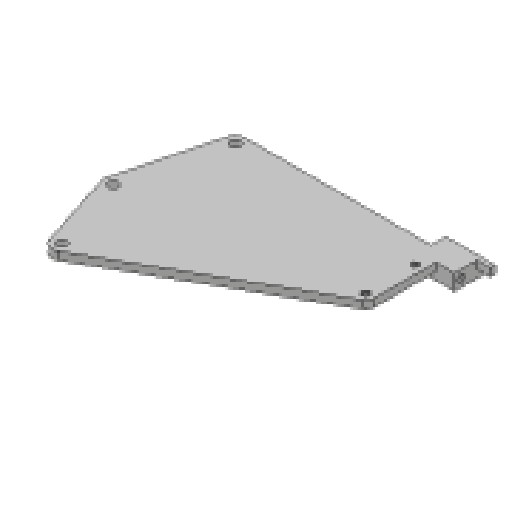
# Autodesk Inventor part: intakeSlidesWheelHolder
Saved by Autodesk Inventor 2023 (Build 270158000, 158)
## iProperties
Created: 2022-11-03
Part Number: intakeSlidesWheelHolder
Material: Generic
Document SubType Name: Modeling
Designer: deli
Density: 1 g/cm^3
Appearance: Default
Author: deli
Autodesk Inventor part; units mm, degrees
ref_plane "YZ Plane" through (0, 0, 0) normal (1, 0, 0) x (0, 1, 0)
ref_plane "XZ Plane" through (0, 0, 0) normal (0, 1, 0) x (-1, 0, 0)
ref_plane "XY Plane" through (0, 0, 0) normal (0, 0, 1) x (1, 0, 0)
sketch "Sketch1" plane through (0, 0, 0) normal (0, 1, 0) x (-1, 0, 0)
  circle A0 centre (23.0548, 41.1652) radius 1.5
  circle A1 centre (23.0548, 21.1652) radius 1.5
  arc A2 (26.5548, 41.1652) -> (19.5548, 41.1652) centre (23.0548, 41.1652) ccw
  line L0 (26.5548, 41.1652) -> (26.5548, 11.1652)
  line L1 (101.8798, 11.1652) -> (12.0548, 11.1652)
  line L2 (19.5548, 16.1652) -> (19.5548, 41.1652)
  line L3 (12.0548, 11.1652) -> (12.0548, 16.1652)
  line L4 (12.0548, 16.1652) -> (19.5548, 16.1652)
  circle A3 centre (112.0548, 54.1652) radius 2
  circle A4 centre (112.0548, 54.1652) radius 25 construction
  circle A5 centre (101.8798, 15.1652) radius 2
  circle A6 centre (101.8798, 85.1652) radius 2
  arc A7 (101.8798, 11.1652) -> (105.7503, 14.1554) centre (101.8798, 15.1652) ccw
  arc A8 (115.9253, 53.1554) -> (115.8554, 55.4126) centre (112.0548, 54.1652) ccw
  arc A9 (105.6804, 86.4126) -> (99.9109, 88.6471) centre (101.8798, 85.1652) ccw
  line L5 (105.7503, 14.1554) -> (115.9253, 53.1554)
  line L6 (115.8554, 55.4126) -> (105.6804, 86.4126)
  line L7 (21.332, 44.2118) -> (99.9109, 88.6471)
  line L8 (12.0548, 11.1652) -> (26.5548, 11.1652)
  line L9 (26.5548, 11.1652) -> (26.5548, 5.1652)
  line L10 (26.5548, 5.1652) -> (11.2902, 5.1652)
  line L11 (12.0548, 7.1652) -> (12.0548, 11.1652)
  line L12 (11.2902, 5.1652) -> (6.7902, 5.1652)
  line L13 (6.7902, 5.1652) -> (6.7902, 7.1652)
  line L14 (6.7902, 7.1652) -> (12.0548, 7.1652)
  point P0 (0, 0)
  dimension "d0" = 3
  dimension "d1" = 2
  dimension "d2" = 20
  dimension "d3" = 10
  dimension "d20" = 11
  dimension "d28" = 4
  dimension "d29" = 85.5
  dimension "d30" = 3.5
  dimension "d32" = 5
  dimension "d33" = 50
  dimension "d34" = 4
  dimension "d35" = 75.325
  dimension "d36" = 75.325
  dimension "d39" = 8
  dimension "d40" = 39
  dimension "d42" = 31
  dimension "d43" = 11
  dimension "d58" = 2
  dimension "d59" = 4.5
  constraints: 30 end point, 10 centre point, 9 point on circle, 9 tangent, 5 coincident, 4 equal radius, 4 horizontal, 4 perpendicular, 3 parallel, 2 collinear, 2 point on line, 1 vertical
  measures "d0" diameter of A0
  measures "d1" radial gap between concentric circles of A2 A0
  measures "d2" distance of A0.centre A1.centre
  measures "d3" distance from line of L1 A1.centre
  measures "d20" distance from line of A1.centre L3
  measures "d28" diameter of A3
  measures "d29" distance from line of L0 A3.centre
  measures "d30" distance from line of A1.centre L0
  measures "d32" distance of L1.end L3.end
  measures "d33" diameter of A4
  measures "d34" diameter of A5
  measures "d35" distance from line of L0 A5.centre
  measures "d36" distance from line of A6.centre L0
  measures "d39" diameter of A7
  measures "d40" vertical distance of A3.centre A5.centre
  measures "d42" vertical distance of A6.centre A3.centre
  measures "d43" distance between parallel lines of L4 L10
  measures "d58" distance of L12.end L13.end
  measures "d59" distance of L10.end L12.end
extrude "Extrusion1" add sketch "Sketch1" along normal blind 3.175
sketch "Sketch2" plane through (0, 3.175, 0) normal (0, 1, 0) x (1, 0, 0)
  line L0 (-19.5548, -16.1652) -> (-12.0548, -16.1652) projected
  line L1 (-6.7902, -5.1652) -> (-26.5548, -5.1652) projected
  line L2 (-12.0548, -16.1652) -> (-26.5548, -16.1652)
  line L3 (-26.5548, -16.1652) -> (-26.5548, -5.1652)
  line L4 (-26.5548, -5.1652) -> (-12.0548, -5.1652)
  line L5 (-12.0548, -5.1652) -> (-12.0548, -16.1652)
  point P0 (0, 0)
  point P1 (-12.0548, -1.1652)
  point P2 (-12.0548, -1.1652)
  constraints: 8 end point, 2 parallel, 1 horizontal, 1 perpendicular, 1 other
extrude "Extrusion2" add sketch "Sketch2" against normal blind 6.35
thread "Thread1" size "M3x0.5" class "6H" standard "ANSI Metric M Profile" full length
thread "Thread3" size "M3x0.5" class "6H" standard "ANSI Metric M Profile" full length
sketch "Sketch5" plane through (-12.0548, 3.175, 16.1652) normal (1, 0, 0) x (0, 0, -1)
  circle A0 centre (2.5, -3.175) radius 1.5
  line L0 (0, 0) -> (9, 0) projected
  line L1 (0, -6.35) -> (0, 0) projected
  point P0 (16.1652, -3.175)
  point P1 (15, 0)
  dimension "d44" = 3
  dimension "d45" = 3.175
  dimension "d47" = 1
  constraints: 1 centre point
  measures "d44" diameter of A0
  measures "d45" distance from line of A0.centre L0
  measures "d47" distance edge to line of A0 L1
extrude "Extrusion5" cut sketch "Sketch5" against normal blind 8
thread "Thread5" size "M3x0.5" class "6H" standard "ANSI Metric M Profile" full length
equation "\"d36\" = d35"
body "Solid1"
